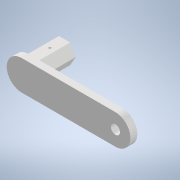
# Autodesk Inventor part: Acople_TransPot
Saved by Autodesk Inventor 2022 (Build 260153000, 153)
## iProperties
Created: 2022-02-22
Part Number: Acople_TransPot
Material: Generic
Document SubType Name: Modeling
Designer: katha
Density: 1 g/cm^3
Appearance: Default
Author: katha
Autodesk Inventor part; units mm, degrees
ref_plane "YZ Plane" through (0, 0, 0) normal (1, 0, 0) x (0, 1, 0)
ref_plane "XZ Plane" through (0, 0, 0) normal (0, 1, 0) x (-1, 0, 0)
ref_plane "XY Plane" through (0, 0, 0) normal (0, 0, 1) x (1, 0, 0)
sketch "Sketch1" plane through (0, 0, 0) normal (0, 0, 1) x (1, 0, 0)
  line L0 (2.8279, 4.8981) -> (-2.8279, 4.8981) projected
  line L1 (-2.8279, 4.8981) -> (-5.6558, 0) projected
  line L2 (-5.6558, 0) -> (-2.8279, -4.8981) projected
  line L3 (-2.8279, -4.8981) -> (2.8279, -4.8981) projected
  line L4 (2.8279, -4.8981) -> (5.6558, 0) projected
  line L5 (5.6558, 0) -> (2.8279, 4.8981) projected
  line L6 (1.6732, 2.8981) -> (3.3464, 0) projected
  line L7 (-1.6732, 2.8981) -> (1.6732, 2.8981) projected
  line L8 (-3.3464, 0) -> (-1.6732, 2.8981) projected
  line L9 (-1.6732, -2.8981) -> (-3.3464, 0) projected
  line L10 (1.6732, -2.8981) -> (-1.6732, -2.8981) projected
  line L11 (3.3464, 0) -> (1.6732, -2.8981) projected
  point P0 (0, 0)
extrude "Extrusion1" add sketch "Sketch1" against normal blind 15
sketch "Sketch2" plane through (0, 0, 0) normal (0, 0, 1) x (1, 0, 0)
  line L0 (2.8279, 4.8981) -> (-2.8279, 4.8981) projected
  line L1 (-2.8279, 4.8981) -> (-5.6558, 0) projected
  line L2 (-5.6558, 0) -> (-2.8279, -4.8981) projected
  line L3 (-2.8279, -4.8981) -> (2.8279, -4.8981) projected
  line L4 (2.8279, -4.8981) -> (5.6558, 0) projected
  line L5 (5.6558, 0) -> (2.8279, 4.8981) projected
  point P0 (0, 0)
extrude "Extrusion2" add sketch "Sketch2" along normal blind 3
sketch "Sketch3" plane through (0, 0, 3) normal (0, 0, 1) x (1, 0, 0)
  circle A0 centre (47, 0) radius 2.3
  circle A1 centre (0, 0) radius 7.5 projected
  circle A2 centre (47, 0) radius 7.5
  line L0 (0, -7.5) -> (47, -7.5)
  line L1 (47, 0) -> (12.3969, 0) construction
  line L2 (0, 7.5) -> (47, 7.5)
  point P0 (0, 0)
  dimension "d13" = 15
  dimension "d5" = 4.6
  dimension "d14" = 47
  constraints: 6 end point, 3 horizontal, 2 symmetric about line, 1 centre point, 1 coincident, 5 other
  measures "d5" diameter of A0
  measures "d14" distance of L0.start L0.end
fillet "Fillet1" radius 1 6 edges at (0, 4.8981, 3) (4.2419, 2.449, 3) (4.2419, -2.449, 3) (0, -4.8981, 3) (-4.2419, -2.449, 3) (-4.2419, 2.449, 3)
sketch "Sketch4" plane through (-2.8279, -4.8981, -15) normal (0, -1, 0) x (1, 0, 0)
  line L0 (0, 17) -> (5.6558, 17) projected
  line L1 (0, 0) -> (0, 17) projected
  line L2 (5.6558, 0) -> (0, 0) projected
  line L3 (5.6558, 0) -> (5.6558, 17) projected
  line L4 (4.5011, 15) -> (1.1547, 15) projected
  line L5 (2.8279, 15) -> (2.8279, 0) construction
  line L6 (1.1547, 0) -> (4.5011, 0) projected
  circle A0 centre (2.8279, 7.5) radius 0.625
  dimension "d10" = 1.25
  constraints: 2 end point, 2 midpoint, 1 centre point
  measures "d10" diameter of A0
extrude "Extrusion4" cut sketch "Sketch4" against normal blind 10 contours A0
extrude "Extrusion5" add sketch "Sketch3" along normal blind 3.5
body "Solid1"
